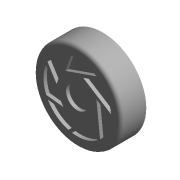
# Autodesk Inventor part: bottom-cap
Saved by Autodesk Inventor 2015 (Build 190159000, 159)
## iProperties
Created: 2014-12-10
Part Number: bottom-cap
Material: Generic
Document SubType Name: Modeling
Designer: Adam
Density: 1 g/cm^3
Appearance: Cyan
Author: Adam
Autodesk Inventor part; units mm, degrees
ref_plane "YZ Plane" through (0, 0, 0) normal (1, 0, 0) x (0, 1, 0)
ref_plane "XZ Plane" through (0, 0, 0) normal (0, 1, 0) x (-1, 0, 0)
ref_plane "XY Plane" through (0, 0, 0) normal (0, 0, 1) x (1, 0, 0)
sketch "Sketch1" plane through (0, 0, 0) normal (0, 0, 1) x (1, 0, 0)
  circle A0 centre (0, 0) radius 6.5 projected
  circle A1 centre (0, 0) radius 5
  point P0 (0, 0)
  dimension "d0" = 1.5
  constraints: 1 centre point, 1 coincident
  measures "d0" radial gap between concentric circles of A0 A1
extrude "Extrusion1" add sketch "Sketch1" against normal blind 2.8
sketch "Sketch2" plane through (0, 0, 0) normal (0, 0, 1) x (1, 0, 0)
  circle A0 centre (0, 0) radius 6.5 projected
  point P0 (0, 0)
extrude "Extrusion2" add sketch "Sketch2" along normal mid plane 2
fillet "Fillet1" radius 0.5 1 edges at (-6.5, 0, 1)
sketch "Sketch3" plane through (0, 0, 1) normal (0, 0, 1) x (1, 0, 0)
  line L0 (-1.7757, 2.5328) -> (2.8763, 4.1461) projected
  arc A0 (2.8763, 4.1461) -> (-0.9181, 4.9618) centre (0, 0) ccw projected
  line L1 (-0.9181, 4.9618) -> (-1.7757, 2.5328) projected
  line L2 (0.8731, 2.9674) -> (5.0349, 0.3362) projected
  arc A1 (5.0349, 0.3362) -> (3.3069, 3.8115) centre (0, 0) ccw projected
  line L3 (3.3069, 3.8115) -> (0.8731, 2.9674) projected
  line L4 (2.8644, 1.1676) -> (3.4021, -3.7268) projected
  arc A2 (3.4021, -3.7268) -> (5.0417, -0.209) centre (0, 0) ccw projected
  line L5 (5.0417, -0.209) -> (2.8644, 1.1676) projected
  circle A3 centre (0, 0) radius 1.682 projected
  line L6 (2.6988, -1.5115) -> (-0.7925, -4.9834) projected
  arc A4 (-0.7925, -4.9834) -> (2.9801, -4.0721) centre (0, 0) ccw projected
  line L7 (2.9801, -4.0721) -> (2.6988, -1.5115) projected
  line L8 (0.5009, -3.0524) -> (-4.3904, -2.4875) projected
  arc A5 (-4.3904, -2.4875) -> (-1.3257, -4.8688) centre (0, 0) ccw projected
  line L9 (-1.3257, -4.8688) -> (0.5009, -3.0524) projected
  line L10 (-2.0741, -2.2947) -> (-4.6821, 1.8816) projected
  arc A6 (-4.6821, 1.8816) -> (-4.6331, -1.9992) centre (0, 0) ccw projected
  line L11 (-4.6331, -1.9992) -> (-2.0741, -2.2947) projected
  line L12 (-3.0873, 0.1909) -> (-1.4482, 4.8338) projected
  arc A7 (-1.4482, 4.8338) -> (-4.4518, 2.3758) centre (0, 0) ccw projected
  line L13 (-4.4518, 2.3758) -> (-3.0873, 0.1909) projected
  point P0 (0, 0)
extrude "Extrusion3" cut sketch "Sketch3" against normal blind 0.5
fillet "Fillet2" radius 1 1 edges at (-5, 0, -1)
body "Solid1"
